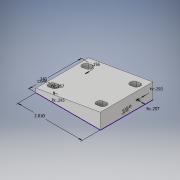
# Autodesk Inventor part: shim 10 Deg
Saved by Autodesk Inventor 2018 (Build 220112000, 112)
## iProperties
Created: 2018-03-27
Part Number: shim 10 Deg
Material: Generic
Document SubType Name: Modeling
Designer: prakh
Density: 1 g/cm^3
Appearance: Default
Author: prakh
Autodesk Inventor part; units mm, degrees
ref_plane "YZ Plane" through (0, 0, 0) normal (1, 0, 0) x (0, 1, 0)
ref_plane "XZ Plane" through (0, 0, 0) normal (0, 1, 0) x (-1, 0, 0)
ref_plane "XY Plane" through (0, 0, 0) normal (0, 0, 1) x (1, 0, 0)
sketch "Sketch1" plane through (0, 0, 0) normal (0, 1, 0) x (-1, 0, 0)
  line L0 (25.527, 20.828) -> (-25.527, 20.828)
  line L1 (-25.527, 20.828) -> (-25.527, -20.828)
  line L2 (-25.527, -20.828) -> (25.527, -20.828)
  line L3 (25.527, -20.828) -> (25.527, 20.828)
  circle A0 centre (18.9992, 13.3858) radius 1.9837
  circle A1 centre (18.9992, -13.3858) radius 1.9837
  circle A2 centre (-18.9992, -13.3858) radius 1.9837
  circle A3 centre (-18.9992, 13.3858) radius 1.9837
  circle A4 centre (18.9992, 13.3858) radius 3.048 construction
  point P0 (0, 0)
  point P1 (25.527, 0)
  point P2 (0, -20.828)
  dimension "d0" = 3.9675
  dimension "d1" = 41.656
  dimension "d2" = 51.054
  dimension "d3" = 6.096
  dimension "d4" = 7.4422
  dimension "d5" = 6.5278
  dimension "d6" = 7.4422
  dimension "d7" = 6.5278
  constraints: 8 end point, 5 centre point, 3 equal radius, 3 horizontal alignment, 3 vertical alignment, 2 midpoint, 2 parallel, 1 coincident, 1 horizontal, 1 perpendicular
  measures "d0" diameter of A1
  measures "d1" distance of L2.end L0.start
  measures "d2" distance of L0.start L0.end
  measures "d3" diameter of A4
  measures "d4" distance from line of L0 A4.centre
  measures "d5" distance from line of A4.centre L3
  measures "d6" distance from line of L2 A2.centre
  measures "d7" distance from line of A2.centre L1
sketch "Sketch10" plane through (0, 0, 0) normal (0, 0, 1) x (1, 0, 0)
  line L0 (-25.527, 0) -> (25.527, 0)
  line L1 (25.527, 0) -> (25.527, 12.1772)
  line L2 (-25.527, 0) -> (-25.527, 3.175)
  line L3 (-25.527, 3.175) -> (25.527, 12.1772)
  point P0 (0, 0)
  dimension "d61" = 10
  dimension "d62" = 3.175
  constraints: 8 end point, 1 horizontal, 1 perpendicular, 1 vertical
  measures "d61" angle of L0 L3
  measures "d62" distance of L0.start L2.end
extrude "Extrusion8" add sketch "Sketch10" along normal mid plane 41.656
sketch "Sketch11" plane through (-25.527, 0, 20.828) normal (0, -1, 0) x (1, 0, 0)
  line L0 (46.1137, -7.4422) -> (42.9387, -7.4422) construction
  line L1 (46.1137, -4.9149) -> (42.9387, -4.9149)
  line L2 (42.9387, -9.9695) -> (46.1137, -9.9695)
  arc A0 (46.1137, -9.9695) -> (46.1137, -4.9149) centre (46.1137, -7.4422) ccw
  arc A1 (42.9387, -4.9149) -> (42.9387, -9.9695) centre (42.9387, -7.4422) ccw
  line L3 (46.1137, -34.2138) -> (42.9387, -34.2138) construction
  line L4 (51.054, -41.656) -> (51.054, 0) projected
  line L5 (46.1137, -36.7411) -> (42.9387, -36.7411)
  line L6 (42.9387, -31.6865) -> (46.1137, -31.6865)
  arc A2 (46.1137, -36.7411) -> (46.1137, -31.6865) centre (46.1137, -34.2138) ccw
  arc A3 (42.9387, -31.6865) -> (42.9387, -36.7411) centre (42.9387, -34.2138) ccw
  line L7 (8.1153, -34.2138) -> (4.9403, -34.2138) construction
  line L8 (8.1153, -36.7411) -> (4.9403, -36.7411)
  line L9 (4.9403, -31.6865) -> (8.1153, -31.6865)
  arc A4 (8.1153, -36.7411) -> (8.1153, -31.6865) centre (8.1153, -34.2138) ccw
  arc A5 (4.9403, -31.6865) -> (4.9403, -36.7411) centre (4.9403, -34.2138) ccw
  line L10 (8.1153, -7.4422) -> (4.9403, -7.4422) construction
  line L11 (8.1153, -9.9695) -> (4.9403, -9.9695)
  line L12 (4.9403, -4.9149) -> (8.1153, -4.9149)
  arc A6 (8.1153, -9.9695) -> (8.1153, -4.9149) centre (8.1153, -7.4422) ccw
  arc A7 (4.9403, -4.9149) -> (4.9403, -9.9695) centre (4.9403, -7.4422) ccw
  point P0 (25.527, -20.828)
  point P1 (44.5262, -7.4422)
  point P2 (44.5262, -34.2138)
  point P3 (6.5278, -34.2138)
  point P4 (6.5278, -7.4422)
  point P5 (44.5262, -7.4422)
  point P6 (44.5262, -34.2138)
  point P7 (6.5278, -34.2138)
  point P8 (6.5278, -7.4422)
  point P9 (44.5262, -9.9695)
  point P10 (6.5278, -36.7411)
  dimension "d65" = 3.175
  dimension "d66" = 2.5273
  constraints: 32 end point, 16 point on circle, 16 tangent, 8 centre point, 8 horizontal alignment, 6 midpoint, 6 vertical alignment, 4 parallel, 4 point on line, 3 equal radius, 1 collinear, 1 horizontal, 1 perpendicular
  measures "d65" distance of L3.start L3.end
  measures "d66" radius of A6
extrude "Extrusion9" cut sketch "Sketch11" against normal blind 41.656
sketch "Sketch13" plane through (25.527, 0, 20.828) normal (1, 0, 0) x (0, 0, -1)
  line L0 (41.656, 12.1772) -> (0, 12.1772) projected
  line L1 (0, 0) -> (0, 12.1772) projected
  line L2 (41.656, 0) -> (0, 0) projected
  line L3 (41.656, 12.1772) -> (41.656, 0) projected
  line L4 (25.4999, 2.032) -> (16.1561, 2.032)
  line L5 (19.4258, 2.032) -> (17.3288, 2.032)
  line L6 (17.3288, 2.032) -> (17.3288, 2.5852)
  line L7 (17.3288, 2.5852) -> (17.9978, 2.5852)
  line L8 (17.9978, 2.5852) -> (17.9978, 4.2653)
  line L9 (17.9978, 4.2653) -> (17.3288, 4.2653)
  line L10 (17.3288, 4.2653) -> (17.3288, 4.7825)
  spline S0 degree 2 poles (17.3288, 4.7825) (17.4755, 4.7825) (17.7662, 4.8211) (17.8537, 4.8622) knots 0 0 0 1 2 2 2
  spline S1 degree 2 poles (17.8537, 4.8622) (17.954, 4.9137) (18.0672, 5.0861) (18.0775, 5.2147) knots 0 0 0 1 2 2 2
  line L11 (18.0775, 5.2147) -> (18.7722, 5.2147)
  line L12 (18.7722, 5.2147) -> (18.7722, 2.5852)
  line L13 (18.7722, 2.5852) -> (19.4258, 2.5852)
  line L14 (19.4258, 2.5852) -> (19.4258, 2.032)
  spline S2 degree 2 poles (22.3074, 3.6195) (22.3074, 3.2078) (22.1762, 2.5903) (22.0296, 2.3819) knots 0 0 0 1 2 2 2
  spline S3 degree 2 poles (22.0296, 2.3819) (21.8855, 2.1761) (21.4198, 1.9651) (21.0853, 1.9651) knots 0 0 0 1 2 2 2
  spline S4 degree 2 poles (21.0853, 1.9651) (20.7482, 1.9651) (20.2851, 2.1761) (20.1385, 2.3871) knots 0 0 0 1 2 2 2
  spline S5 degree 2 poles (20.1385, 2.3871) (19.9918, 2.5955) (19.8606, 3.2078) (19.8606, 3.6195) knots 0 0 0 1 2 2 2
  spline S6 degree 2 poles (19.8606, 3.6195) (19.8606, 4.0415) (19.9918, 4.6384) (20.141, 4.8545) knots 0 0 0 1 2 2 2
  spline S7 degree 2 poles (20.141, 4.8545) (20.2903, 5.0655) (20.7611, 5.2713) (21.0853, 5.2713) knots 0 0 0 1 2 2 2
  spline S8 degree 2 poles (21.0853, 5.2713) (21.4275, 5.2713) (21.8855, 5.0552) (22.0321, 4.8416) knots 0 0 0 1 2 2 2
  spline S9 degree 2 poles (22.0321, 4.8416) (22.1762, 4.6332) (22.3074, 4.0183) (22.3074, 3.6195) knots 0 0 0 1 2 2 2
  spline S10 degree 2 poles (21.5073, 3.6195) (21.5073, 4.2087) (21.3143, 4.6847) (21.0853, 4.6847) knots 0 0 0 1 2 2 2
  spline S11 degree 2 poles (21.0853, 4.6847) (20.8563, 4.6847) (20.6608, 4.2087) (20.6608, 3.6169) knots 0 0 0 1 2 2 2
  spline S12 degree 2 poles (20.6608, 3.6169) (20.6608, 3.0354) (20.8563, 2.5517) (21.0853, 2.5517) knots 0 0 0 1 2 2 2
  spline S13 degree 2 poles (21.0853, 2.5517) (21.3117, 2.5517) (21.5073, 3.0354) (21.5073, 3.6195) knots 0 0 0 1 2 2 2
  spline S14 degree 2 poles (24.4738, 4.4145) (24.4738, 4.0518) (23.9696, 3.5552) (23.6093, 3.5552) knots 0 0 0 1 2 2 2
  spline S15 degree 2 poles (23.6093, 3.5552) (23.2466, 3.5552) (22.7423, 4.0518) (22.7423, 4.4145) knots 0 0 0 1 2 2 2
  spline S16 degree 2 poles (22.7423, 4.4145) (22.7423, 4.7773) (23.2466, 5.2739) (23.6093, 5.2739) knots 0 0 0 1 2 2 2
  spline S17 degree 2 poles (23.6093, 5.2739) (23.9721, 5.2739) (24.4738, 4.7773) (24.4738, 4.4145) knots 0 0 0 1 2 2 2
  spline S18 degree 2 poles (24.0081, 4.4145) (24.0081, 4.5818) (23.7792, 4.8211) (23.6093, 4.8211) knots 0 0 0 1 2 2 2
  spline S19 degree 2 poles (23.6093, 4.8211) (23.4395, 4.8211) (23.208, 4.5844) (23.208, 4.4145) knots 0 0 0 1 2 2 2
  spline S20 degree 2 poles (23.208, 4.4145) (23.208, 4.2396) (23.4421, 4.008) (23.6093, 4.008) knots 0 0 0 1 2 2 2
  spline S21 degree 2 poles (23.6093, 4.008) (23.7792, 4.008) (24.0081, 4.2447) (24.0081, 4.4145) knots 0 0 0 1 2 2 2
  point P0 (20.828, 0)
  point P1 (20.828, 0)
  point P2 (20.828, 2.032)
  dimension "d69" = 2.032
  constraints: 2 end point, 2 horizontal, 2 midpoint, 1 vertical alignment
  measures "d69" distance between parallel lines of L2 L4
extrude "Extrusion10" cut sketch "Sketch13" against normal blind 0.381 contours S4 S5 S6 S7 S8 S9 S2 S3 L4 | L4 S3 S4 | L4 L6 L7 L8 L9 L10 S0 S1 L11 L12 L13 L14 | S14 S15 S16 S17
equation "\"d6\" = d4"
equation "\"d7\" = d5"
equation "\"d23\" = d22"
equation "\"d25\" = 0.5 * d24"
equation "\"d22\" = 3.175"
equation "\"d24\" = 4.7625"
body "Solid2"
